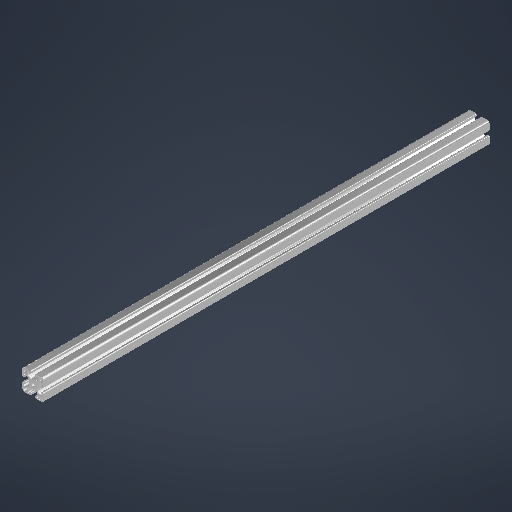
# Autodesk Inventor part: profileAluAvant1
Saved by Autodesk Inventor 2026.2 (Build 302298010, 298A)
## iProperties
Part Number: profileAluAvant1
Material: Générique
Document SubType Name: Modélisation
Designer: quent
Appearance: Aluminium - Plat
Author: quent
Autodesk Inventor part; units mm, degrees
ref_plane "Plan YZ" through (0, 0, 0) normal (1, 0, 0) x (0, 1, 0)
ref_plane "Plan XZ" through (0, 0, 0) normal (0, 1, 0) x (-1, 0, 0)
ref_plane "Plan XY" through (0, 0, 0) normal (0, 0, 1) x (1, 0, 0)
sketch "Esquisse1" plane through (0, 0, 0) normal (0, 0, 1) x (1, 0, 0)
  arc A0 (-11.4345, 5.1437) -> (-10.3095, 4.0187) centre (-10.3095, 5.1437) ccw
  line L0 (-8.8095, 4.0187) -> (-10.3095, 4.0187)
  arc A1 (-8.8095, 4.0187) -> (-8.0595, 4.7687) centre (-8.8095, 4.7687) ccw
  line L1 (-8.0595, 5.8937) -> (-8.0595, 4.7687)
  arc A2 (-8.0595, 5.8937) -> (-8.4345, 6.2687) centre (-8.4345, 5.8937) ccw
  line L2 (-9.5595, 6.2687) -> (-8.4345, 6.2687)
  arc A3 (-9.9345, 6.6437) -> (-9.5595, 6.2687) centre (-9.5595, 6.6437) ccw
  arc A4 (-8.0595, 8.5187) -> (-9.9345, 6.6437) centre (-8.0595, 6.6437) ccw
  line L3 (-7.0788, 8.5187) -> (-8.0595, 8.5187)
  arc A5 (-4.4272, 7.4204) -> (-7.0788, 8.5187) centre (-7.0788, 4.7687) ccw
  line L4 (-3.3454, 6.3386) -> (-4.4272, 7.4204)
  arc A6 (-2.247, 3.6869) -> (-3.3454, 6.3386) centre (-5.997, 3.6869) ccw
  line L5 (-2.247, -1.6495) -> (-2.247, 3.6869)
  arc A7 (-3.3454, -4.3011) -> (-2.247, -1.6495) centre (-5.997, -1.6495) ccw
  line L6 (-4.4272, -5.3829) -> (-3.3454, -4.3011)
  arc A8 (-7.0788, -6.4813) -> (-4.4272, -5.3829) centre (-7.0788, -2.7313) ccw
  line L7 (-8.0595, -6.4813) -> (-7.0788, -6.4813)
  arc A9 (-9.9345, -4.6063) -> (-8.0595, -6.4813) centre (-8.0595, -4.6063) ccw
  arc A10 (-9.5595, -4.2313) -> (-9.9345, -4.6063) centre (-9.5595, -4.6063) ccw
  line L8 (-8.4345, -4.2313) -> (-9.5595, -4.2313)
  arc A11 (-8.4345, -4.2313) -> (-8.0595, -3.8563) centre (-8.4345, -3.8563) ccw
  line L9 (-8.0595, -2.7313) -> (-8.0595, -3.8563)
  arc A12 (-8.0595, -2.7313) -> (-8.8095, -1.9813) centre (-8.8095, -2.7313) ccw
  line L10 (-10.3095, -1.9813) -> (-8.8095, -1.9813)
  arc A13 (-10.3095, -1.9813) -> (-11.4345, -3.1063) centre (-10.3095, -3.1063) ccw
  line L11 (-11.4345, -10.9813) -> (-11.4345, -3.1063)
  arc A14 (-11.4345, -10.9813) -> (-8.4345, -13.9813) centre (-8.4345, -10.9813) ccw
  line L12 (-0.5595, -13.9813) -> (-8.4345, -13.9813)
  arc A15 (-0.5595, -13.9813) -> (0.5655, -12.8563) centre (-0.5595, -12.8563) ccw
  line L13 (0.5655, -11.3563) -> (0.5655, -12.8563)
  arc A16 (0.5655, -11.3563) -> (-0.1845, -10.6063) centre (-0.1845, -11.3563) ccw
  line L14 (-1.3095, -10.6063) -> (-0.1845, -10.6063)
  arc A17 (-1.3095, -10.6063) -> (-1.6845, -10.9813) centre (-1.3095, -10.9813) ccw
  line L15 (-1.6845, -12.1063) -> (-1.6845, -10.9813)
  arc A18 (-2.0595, -12.4813) -> (-1.6845, -12.1063) centre (-2.0595, -12.1063) ccw
  arc A19 (-3.9345, -10.6063) -> (-2.0595, -12.4813) centre (-2.0595, -10.6063) ccw
  line L16 (-3.9345, -9.6256) -> (-3.9345, -10.6063)
  arc A20 (-2.8362, -6.9739) -> (-3.9345, -9.6256) centre (-0.1845, -9.6256) ccw
  line L17 (-1.7544, -5.8921) -> (-2.8362, -6.9739)
  arc A21 (0.8973, -4.7938) -> (-1.7544, -5.8921) centre (0.8973, -8.5438) ccw
  line L18 (6.2337, -4.7938) -> (0.8973, -4.7938)
  arc A22 (8.8853, -5.8921) -> (6.2337, -4.7938) centre (6.2337, -8.5438) ccw
  line L19 (9.9671, -6.9739) -> (8.8853, -5.8921)
  arc A23 (11.0655, -9.6256) -> (9.9671, -6.9739) centre (7.3155, -9.6256) ccw
  line L20 (11.0655, -10.6063) -> (11.0655, -9.6256)
  arc A24 (9.1905, -12.4813) -> (11.0655, -10.6063) centre (9.1905, -10.6063) ccw
  arc A25 (8.8155, -12.1063) -> (9.1905, -12.4813) centre (9.1905, -12.1063) ccw
  line L21 (8.8155, -10.9813) -> (8.8155, -12.1063)
  arc A26 (8.8155, -10.9813) -> (8.4405, -10.6063) centre (8.4405, -10.9813) ccw
  line L22 (7.3155, -10.6063) -> (8.4405, -10.6063)
  arc A27 (7.3155, -10.6063) -> (6.5655, -11.3563) centre (7.3155, -11.3563) ccw
  line L23 (6.5655, -12.8563) -> (6.5655, -11.3563)
  arc A28 (6.5655, -12.8563) -> (7.6905, -13.9813) centre (7.6905, -12.8563) ccw
  line L24 (15.5655, -13.9813) -> (7.6905, -13.9813)
  arc A29 (15.5655, -13.9813) -> (18.5655, -10.9813) centre (15.5655, -10.9813) ccw
  line L25 (18.5655, -3.1063) -> (18.5655, -10.9813)
  arc A30 (18.5655, -3.1063) -> (17.4405, -1.9813) centre (17.4405, -3.1063) ccw
  line L26 (15.9405, -1.9813) -> (17.4405, -1.9813)
  arc A31 (15.9405, -1.9813) -> (15.1905, -2.7313) centre (15.9405, -2.7313) ccw
  line L27 (15.1905, -3.8563) -> (15.1905, -2.7313)
  arc A32 (15.1905, -3.8563) -> (15.5655, -4.2313) centre (15.5655, -3.8563) ccw
  line L28 (16.6905, -4.2313) -> (15.5655, -4.2313)
  arc A33 (17.0655, -4.6063) -> (16.6905, -4.2313) centre (16.6905, -4.6063) ccw
  arc A34 (15.1905, -6.4813) -> (17.0655, -4.6063) centre (15.1905, -4.6063) ccw
  line L29 (14.2098, -6.4813) -> (15.1905, -6.4813)
  arc A35 (11.5581, -5.3829) -> (14.2098, -6.4813) centre (14.2098, -2.7313) ccw
  line L30 (10.4763, -4.3011) -> (11.5581, -5.3829)
  arc A36 (9.378, -1.6495) -> (10.4763, -4.3011) centre (13.128, -1.6495) ccw
  line L31 (9.378, 3.6869) -> (9.378, -1.6495)
  arc A37 (10.4763, 6.3386) -> (9.378, 3.6869) centre (13.128, 3.6869) ccw
  line L32 (11.5581, 7.4204) -> (10.4763, 6.3386)
  arc A38 (14.2098, 8.5187) -> (11.5581, 7.4204) centre (14.2098, 4.7687) ccw
  line L33 (15.1905, 8.5187) -> (14.2098, 8.5187)
  arc A39 (17.0655, 6.6437) -> (15.1905, 8.5187) centre (15.1905, 6.6437) ccw
  arc A40 (16.6905, 6.2687) -> (17.0655, 6.6437) centre (16.6905, 6.6437) ccw
  line L34 (15.5655, 6.2687) -> (16.6905, 6.2687)
  arc A41 (15.5655, 6.2687) -> (15.1905, 5.8937) centre (15.5655, 5.8937) ccw
  line L35 (15.1905, 4.7687) -> (15.1905, 5.8937)
  arc A42 (15.1905, 4.7687) -> (15.9405, 4.0187) centre (15.9405, 4.7687) ccw
  line L36 (17.4405, 4.0187) -> (15.9405, 4.0187)
  arc A43 (17.4405, 4.0187) -> (18.5655, 5.1437) centre (17.4405, 5.1437) ccw
  line L37 (18.5655, 13.0187) -> (18.5655, 5.1437)
  arc A44 (18.5655, 13.0187) -> (15.5655, 16.0187) centre (15.5655, 13.0187) ccw
  line L38 (7.6905, 16.0187) -> (15.5655, 16.0187)
  arc A45 (7.6905, 16.0187) -> (6.5655, 14.8937) centre (7.6905, 14.8937) ccw
  line L39 (6.5655, 13.3937) -> (6.5655, 14.8937)
  arc A46 (6.5655, 13.3937) -> (7.3155, 12.6437) centre (7.3155, 13.3937) ccw
  line L40 (8.4405, 12.6437) -> (7.3155, 12.6437)
  arc A47 (8.4405, 12.6437) -> (8.8155, 13.0187) centre (8.4405, 13.0187) ccw
  line L41 (8.8155, 14.1437) -> (8.8155, 13.0187)
  arc A48 (9.1905, 14.5187) -> (8.8155, 14.1437) centre (9.1905, 14.1437) ccw
  arc A49 (11.0655, 12.6437) -> (9.1905, 14.5187) centre (9.1905, 12.6437) ccw
  line L42 (11.0655, 11.663) -> (11.0655, 12.6437)
  arc A50 (9.9671, 9.0114) -> (11.0655, 11.663) centre (7.3155, 11.663) ccw
  line L43 (8.8853, 7.9296) -> (9.9671, 9.0114)
  arc A51 (6.2337, 6.8312) -> (8.8853, 7.9296) centre (6.2337, 10.5812) ccw
  line L44 (0.8973, 6.8312) -> (6.2337, 6.8312)
  arc A52 (-1.7544, 7.9296) -> (0.8973, 6.8312) centre (0.8973, 10.5812) ccw
  line L45 (-2.8362, 9.0114) -> (-1.7544, 7.9296)
  arc A53 (-3.9345, 11.663) -> (-2.8362, 9.0114) centre (-0.1845, 11.663) ccw
  line L46 (-3.9345, 12.6437) -> (-3.9345, 11.663)
  arc A54 (-2.0595, 14.5187) -> (-3.9345, 12.6437) centre (-2.0595, 12.6437) ccw
  arc A55 (-1.6845, 14.1437) -> (-2.0595, 14.5187) centre (-2.0595, 14.1437) ccw
  line L47 (-1.6845, 13.0187) -> (-1.6845, 14.1437)
  arc A56 (-1.6845, 13.0187) -> (-1.3095, 12.6437) centre (-1.3095, 13.0187) ccw
  line L48 (-0.1845, 12.6437) -> (-1.3095, 12.6437)
  arc A57 (-0.1845, 12.6437) -> (0.5655, 13.3937) centre (-0.1845, 13.3937) ccw
  line L49 (0.5655, 14.8937) -> (0.5655, 13.3937)
  arc A58 (0.5655, 14.8937) -> (-0.5595, 16.0187) centre (-0.5595, 14.8937) ccw
  line L50 (-8.4345, 16.0187) -> (-0.5595, 16.0187)
  arc A59 (-8.4345, 16.0187) -> (-11.4345, 13.0187) centre (-8.4345, 13.0187) ccw
  line L51 (-11.4345, 5.1437) -> (-11.4345, 13.0187)
  line L52 (12.4155, -12.2563) -> (12.4155, -8.2063)
  arc A60 (12.7905, -7.8313) -> (12.4155, -8.2063) centre (12.7905, -8.2063) ccw
  line L53 (12.7905, -7.8313) -> (16.8405, -7.8313)
  arc A61 (17.2155, -8.2063) -> (16.8405, -7.8313) centre (16.8405, -8.2063) ccw
  line L54 (17.2155, -8.2063) -> (17.2155, -10.9813)
  arc A62 (15.5655, -12.6313) -> (17.2155, -10.9813) centre (15.5655, -10.9813) ccw
  line L55 (15.5655, -12.6313) -> (12.7905, -12.6313)
  arc A63 (12.4155, -12.2563) -> (12.7905, -12.6313) centre (12.7905, -12.2563) ccw
  line L56 (-9.7095, -7.8313) -> (-5.6595, -7.8313)
  arc A64 (-5.2845, -8.2063) -> (-5.6595, -7.8313) centre (-5.6595, -8.2063) ccw
  line L57 (-5.2845, -8.2063) -> (-5.2845, -12.2563)
  arc A65 (-5.6595, -12.6313) -> (-5.2845, -12.2563) centre (-5.6595, -12.2563) ccw
  line L58 (-5.6595, -12.6313) -> (-8.4345, -12.6313)
  arc A66 (-10.0845, -10.9813) -> (-8.4345, -12.6313) centre (-8.4345, -10.9813) ccw
  line L59 (-10.0845, -10.9813) -> (-10.0845, -8.2063)
  arc A67 (-9.7095, -7.8313) -> (-10.0845, -8.2063) centre (-9.7095, -8.2063) ccw
  line L60 (-5.2845, 14.2937) -> (-5.2845, 10.2437)
  arc A68 (-5.6595, 9.8687) -> (-5.2845, 10.2437) centre (-5.6595, 10.2437) ccw
  line L61 (-5.6595, 9.8687) -> (-9.7095, 9.8687)
  arc A69 (-10.0845, 10.2437) -> (-9.7095, 9.8687) centre (-9.7095, 10.2437) ccw
  line L62 (-10.0845, 10.2437) -> (-10.0845, 13.0187)
  arc A70 (-8.4345, 14.6687) -> (-10.0845, 13.0187) centre (-8.4345, 13.0187) ccw
  line L63 (-8.4345, 14.6687) -> (-5.6595, 14.6687)
  arc A71 (-5.2845, 14.2937) -> (-5.6595, 14.6687) centre (-5.6595, 14.2937) ccw
  line L64 (16.8405, 9.8687) -> (12.7905, 9.8687)
  arc A72 (12.4155, 10.2437) -> (12.7905, 9.8687) centre (12.7905, 10.2437) ccw
  line L65 (12.4155, 10.2437) -> (12.4155, 14.2937)
  arc A73 (12.7905, 14.6687) -> (12.4155, 14.2937) centre (12.7905, 14.2937) ccw
  line L66 (12.7905, 14.6687) -> (15.5655, 14.6687)
  arc A74 (17.2155, 13.0187) -> (15.5655, 14.6687) centre (15.5655, 13.0187) ccw
  line L67 (17.2155, 13.0187) -> (17.2155, 10.2437)
  arc A75 (16.8405, 9.8687) -> (17.2155, 10.2437) centre (16.8405, 10.2437) ccw
  circle A76 centre (3.5655, 1.0187) radius 2.55
  point P0 (0, 0)
  point P1 (0.6155, 4.7687)
  constraints: 152 point on circle, 136 end point, 77 centre point
extrude "Extrusion1" add sketch "Esquisse1" along normal blind 632
